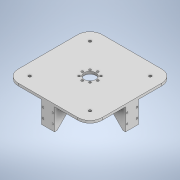
# Autodesk Inventor part: 移動升降板
Saved by Autodesk Inventor 2021 (Build 250183000, 183)
## iProperties
Created: 2023-02-06
Part Number: 移動升降板
Material: 一般
Document SubType Name: Modeling
Designer: brian
Density: 1 g/cm^3
Appearance: 預設
Author: brian
Autodesk Inventor part; units mm, degrees
note: some values were not read from the file. Chosen so that the rebuilt part matches the saved one: direction of "孔3"; direction of "孔5".
ref_plane "YZ Plane" through (0, 0, 0) normal (1, 0, 0) x (0, 1, 0)
ref_plane "XZ Plane" through (0, 0, 0) normal (0, 1, 0) x (-1, 0, 0)
ref_plane "XY Plane" through (0, 0, 0) normal (0, 0, 1) x (1, 0, 0)
sketch "草圖1" plane through (0, 0, 0) normal (0, 1, 0) x (-1, 0, 0)
  line L0 (87, 87) -> (-87, 87)
  line L1 (-87, 87) -> (-87, -87)
  line L2 (-87, -87) -> (87, -87)
  line L3 (87, -87) -> (87, 87)
  line L4 (87, 87) -> (-87, -87) construction
  line L5 (-87, 87) -> (87, -87) construction
  point P0 (0, 0)
  dimension "d0" = 174
  dimension "d1" = 174
  constraints: 12 end point, 2 midpoint, 2 parallel, 1 horizontal, 1 perpendicular
  measures "d0" distance of L2.end L1.end
  measures "d1" distance of L1.end L0.end
extrude "擠出1" add sketch "草圖1" along normal blind 5
sketch "草圖2" plane through (0, 0, 0) normal (0, -1, 0) x (1, 0, 0)
  circle A0 centre (0, 0) radius 12.1
  dimension "d4" = 24.2
  constraints: 1 centre point, 1 coincident
  measures "d4" diameter of A0
extrude "擠出2" cut sketch "草圖2" against normal through all
sketch "草圖3" plane through (0, 0, 0) normal (0, -1, 0) x (1, 0, 0)
  point P0 (0, 0)
  point P1 (16, 0)
  dimension "d7" = 16
  constraints: 1 horizontal alignment
  measures "d7" distance of point (0, 0) point (16, 0)
hole "孔1" at (16, 0, 0) direction (0, 1, 0) diameter 4.5 end through all
pattern_circular "環形陣列1" count 8 over 360 about axis through (0, 0, 0) along (0, 1, 0) of "孔1"
fillet "圓角1" radius 25 4 edges at (87, 2.5, -87) (-87, 2.5, -87) (-87, 2.5, 87) (87, 2.5, 87)
sketch "草圖4" plane through (0, 0, 0) normal (0, -1, 0) x (1, 0, 0)
  circle A0 centre (11.3137, 11.3137) radius 2.25 projected
  circle A1 centre (0, 16) radius 2.25 projected
  circle A2 centre (-11.3137, 11.3137) radius 2.25 projected
  circle A3 centre (-16, 0) radius 2.25 projected
  circle A4 centre (-11.3137, -11.3137) radius 2.25 projected
  circle A5 centre (0, -16) radius 2.25 projected
  circle A6 centre (11.3137, -11.3137) radius 2.25 projected
  circle A7 centre (16, 0) radius 2.25 projected
  circle A8 centre (0, 0) radius 12.1 projected
  arc A9 (87, 62) -> (62, 87) centre (62, 62) ccw projected
  line L0 (-62, 87) -> (62, 87) projected
  arc A10 (-62, 87) -> (-87, 62) centre (-62, 62) ccw projected
  line L1 (-87, -62) -> (-87, 62) projected
  arc A11 (-87, -62) -> (-62, -87) centre (-62, -62) ccw projected
  line L2 (62, -87) -> (-62, -87) projected
  arc A12 (62, -87) -> (87, -62) centre (62, -62) ccw projected
  line L3 (87, 62) -> (87, -62) projected
  line L4 (-62, 87) -> (62, 87) projected
  line L5 (13.5, 87) -> (-13.5, 87)
  line L6 (-13.5, 87) -> (-13.5, 82)
  line L7 (-13.5, 82) -> (13.5, 82)
  line L8 (13.5, 82) -> (13.5, 87)
  line L9 (87, 62) -> (87, -62) projected
  line L10 (87, 13.5) -> (82, 13.5)
  line L11 (82, 13.5) -> (82, -13.5)
  line L12 (82, -13.5) -> (87, -13.5)
  line L13 (87, -13.5) -> (87, 13.5)
  line L14 (62, -87) -> (-62, -87) projected
  line L15 (13.5, -87) -> (-13.5, -87)
  line L16 (-13.5, -87) -> (-13.5, -82)
  line L17 (-13.5, -82) -> (13.5, -82)
  line L18 (13.5, -82) -> (13.5, -87)
  point P0 (0, 82)
  point P1 (82, 0)
  point P2 (0, -82)
  dimension "d19" = 27
  dimension "d20" = 5
  dimension "d21" = 27
  dimension "d22" = 27
  dimension "d23" = 5
  dimension "d24" = 5
  constraints: 24 end point, 6 parallel, 3 horizontal, 3 midpoint, 3 perpendicular, 3 point on line, 2 vertical alignment, 1 horizontal alignment
  measures "d19" distance of L6.end L7.end
  measures "d20" distance of L7.end L5.start
  measures "d21" distance of L10.end L11.end
  measures "d22" distance of L16.end L17.end
  measures "d23" distance of L17.end L15.start
  measures "d24" distance of L11.end L12.end
extrude "擠出3" add sketch "草圖4" along normal blind 45 contours L3 L12 L11 L10 | L8 L7 L6 L0 | L2 L16 L17 L18
chamfer "倒角1" distance 45 angle 45 3 edges at (0, 0, 82) (0, 0, -82) (82, 0, 0)
sketch "草圖6" plane through (-62, 5, 87) normal (0, 0, 1) x (1, 0, 0)
  line L0 (124, 0) -> (124, -5) projected
  line L1 (0, 0) -> (124, 0) projected
  line L2 (0, -5) -> (0, 0) projected
  line L3 (0, -5) -> (48.5, -5) projected
  line L4 (48.5, -5) -> (48.5, -50) projected
  line L5 (75.5, -50) -> (48.5, -50) projected
  line L6 (75.5, -5) -> (75.5, -50) projected
  line L7 (75.5, -5) -> (124, -5) projected
  line L8 (52, -17.3) -> (72, -17.3) construction
  line L9 (72, -17.3) -> (72, -37.3) construction
  line L10 (72, -37.3) -> (52, -37.3) construction
  line L11 (52, -37.3) -> (52, -17.3) construction
  point P0 (62, -5)
  point P1 (62, -37.3)
  point P2 (62, -50)
  dimension "d31" = 20
  dimension "d32" = 20
  dimension "d34" = 12.7
  constraints: 8 end point, 4 coincident, 2 midpoint, 2 parallel, 1 horizontal, 1 perpendicular, 1 vertical alignment
  measures "d31" distance of L9.end L10.end
  measures "d32" distance of L8.end L9.end
  measures "d34" distance between parallel lines of L5 L10
hole "孔2" at (-10, -12.3, 87) at (10, -12.3, 87) at (10, -32.3, 87) at (-10, -32.3, 87) direction (0, 0, -1) diameter 3.3 depth 8
sketch "草圖7" plane through (-10, -32.3, 79) normal (0, 0, 1) x (1, 0, 0)
  circle A0 centre (0, 20) radius 1.65 projected
  circle A1 centre (20, 20) radius 1.65 projected
  circle A2 centre (20, 0) radius 1.65 projected
  circle A3 centre (0, 0) radius 1.65 projected
  circle A4 centre (20, 0) radius 1.65 projected
  circle A5 centre (0, 0) radius 1.65 projected
  point P0 (10, 32.3)
  constraints: 4 coincident
hole "孔3" at (-10, -12.3, 79) at (10, -12.3, 79) at (10, -32.3, 79) at (-10, -32.3, 79) direction (0, 0, -1) diameter 5.5 end up to surface
mirror "鏡射1" about plane through (0, 0, 0) normal (0, 0, 1) of "孔3", "孔2"
sketch "草圖8" plane through (87, 0, 62) normal (1, 0, 0) x (0, 0, -1)
  line L0 (0, 0) -> (0, 5) projected
  line L1 (0, 0) -> (48.5, 0) projected
  line L2 (48.5, 0) -> (48.5, -45) projected
  line L3 (75.5, -45) -> (48.5, -45) projected
  line L4 (75.5, 0) -> (75.5, -45) projected
  line L5 (75.5, 0) -> (124, 0) projected
  line L6 (124, 5) -> (124, 0) projected
  line L7 (0, 5) -> (124, 5) projected
  line L8 (52, -12.3) -> (72, -12.3) construction
  line L9 (72, -12.3) -> (72, -32.3) construction
  line L10 (72, -32.3) -> (52, -32.3) construction
  line L11 (52, -32.3) -> (52, -12.3) construction
  point P0 (62, 0)
  point P1 (62, -12.3)
  point P2 (62, -45)
  dimension "d49" = 20
  dimension "d50" = 20
  dimension "d51" = 12.7
  constraints: 8 end point, 4 coincident, 2 midpoint, 2 parallel, 1 horizontal, 1 perpendicular, 1 vertical alignment
  measures "d49" distance of L9.end L10.end
  measures "d50" distance of L8.end L9.end
  measures "d51" distance from line of point (62, -45) L10
hole "孔4" at (87, -12.3, 10) at (87, -32.3, 10) at (87, -32.3, -10) at (87, -12.3, -10) direction (-1, 0, 0) diameter 3.3 depth 8
sketch "草圖9" plane through (79, -12.3, 10) normal (1, 0, 0) x (0, 0, -1)
  circle A0 centre (0, 0) radius 1.65 projected
  circle A1 centre (20, 0) radius 1.65 projected
  circle A2 centre (20, -20) radius 1.65 projected
  circle A3 centre (0, -20) radius 1.65 projected
  circle A4 centre (0, 0) radius 1.65 projected
  circle A5 centre (0, -20) radius 1.65 projected
  circle A6 centre (20, 0) radius 1.65 projected
  point P0 (10, 12.3)
  constraints: 4 coincident
hole "孔5" at (79, -12.3, 10) at (79, -32.3, 10) at (79, -32.3, -10) at (79, -12.3, -10) direction (-1, 0, 0) diameter 5.5 end up to surface
sketch "草圖10" plane through (0, 5, 0) normal (0, 1, 0) x (1, 0, 0)
  line L0 (62.5, 62.5) -> (-62.5, 62.5)
  line L1 (-62.5, 62.5) -> (-62.5, -62.5)
  line L2 (-62.5, -62.5) -> (62.5, -62.5)
  line L3 (62.5, -62.5) -> (62.5, 62.5)
  circle A0 centre (0, 0) radius 12.1 projected
  line L4 (62.5, 62.5) -> (-62.5, -62.5) construction
  line L5 (-62.5, 62.5) -> (62.5, -62.5) construction
  dimension "d66" = 125
  dimension "d67" = 125
  constraints: 12 end point, 4 coincident, 2 midpoint, 2 parallel, 1 horizontal, 1 perpendicular
  measures "d66" distance of L2.end L1.end
  measures "d67" distance of L1.end L0.end
hole "孔6" at (62.5, 5, -62.5) at (-62.5, 5, -62.5) at (-62.5, 5, 62.5) at (62.5, 5, 62.5) direction (0, -1, 0) diameter 5.5 end through all
equation "\"d0\" = d1"
equation "\"d21\" = d19"
equation "\"d22\" = d19"
equation "\"d23\" = d20"
equation "\"d24\" = d20"
